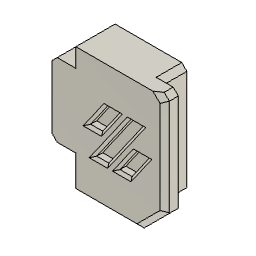
v0.2 Formbot Deck Chain Gap Cover v9 (Autodesk Fusion 360 design; units mm, degrees)
Autodesk Fusion 360 part; units mm, degrees
sketch "Base dimensions" plane through (0, 0, 0) normal (0, 1, 0) x (1, 0, 0)
  line L0 (-15, -8) -> (-6.6, -8)
  line L1 (-6.6, -8) -> (-6.6, 5)
  line L2 (-6.6, 5) -> (-15, 5)
  line L3 (-15, 5) -> (-15, -8)
  line L4 (-17.8, -5.8) -> (-15, -5.8)
  line L5 (-15, -5.8) -> (-15, 2.8)
  line L6 (-15, 2.8) -> (-17.8, 2.8)
  line L7 (-17.8, 2.8) -> (-17.8, -5.8)
  line L8 (-15.0127, 7) -> (-4.6, 7)
  line L9 (-4.6, 7) -> (-4.6, -8)
  line L10 (-4.6, -8) -> (-15.0127, -8)
  line L11 (-15.0127, -8) -> (-15.0127, 7)
  dimension "d1" = 8.4
  dimension "d2" = 13
  dimension "d3" = 2.2
  dimension "d4" = 2.2
  dimension "d5" = 2
  dimension "d6" = 2
  dimension "d21" = 2.8
  constraint horizontal L0
  constraint vertical L1
  constraint horizontal L2
  constraint vertical L3
  constraint horizontal L4
  constraint vertical L5
  constraint horizontal L6
  constraint vertical L7
  constraint coincident L3 L5.end
  constraint horizontal L8
  constraint vertical L9
  constraint horizontal L10
  constraint vertical L11
  measures "d1" distance of L0.start L0.end
  measures "d2" distance of L0.start L2.end
  measures "d3" distance of L0 L4
  measures "d4" distance of L2 L6
  measures "d5" distance of L0.end L9.end
  measures "d6" distance of L1.end L8
  measures "d21" distance of L3 L7
extrude "Extrude1" add sketch "Base dimensions" along normal blind 3 contours L0 L1 L2 L3 L5 L10 | L4 L6 L7 L11 makes body 1 at (-12.2, 0, 3.6667) makes body 2 at (-17.8, 1, 0.0667)
extrude "Extrude2" add sketch "Base dimensions" against normal blind 1.6 contours L0 L1 L2 L3 L5 L10 | L4 L6 L7 L11 bodies 1 2
extrude "Extrude3" add sketch "Base dimensions" against normal blind 1.6 contours L1 L2 L3 L6 L8 L9 L10 L11 bodies 1 2
chamfer "Chamfer1" distance 0.6 angle 45 6 edges at (-6.6, 1.5, -5) (-15, 1.5, -5) (-6.6, 1.5, 8) (-15, 0.7, 8) (-17.8, 0.7, 5.8) (-17.8, 0.7, -2.8) on bodies 1 2
chamfer "Chamfer2" distance 0.6 angle 45 3 edges at (-4.6, -0.8, 8) (-4.6, -0.8, -7) (-15.0127, -0.8, -7) on bodies 1
extrude "Extrude4" add 1 faces at (-15.9418, -1.6, 0.2667) along direction (0, -1, 0) blind 0.004 on bodies 1 bodies 1
extrude "Extrude5" cut 1 faces at (-15.9418, -1.604, 0.2667) along direction (0, 1, 0) up to surface (0.004 mm away) on bodies 1 bodies 1
chamfer "Chamfer3" distance 0.55 distance2 0.55 7 edges at (-14.7127, -1.6, -6.7) (-9.8064, -1.6, -7) (-4.9, -1.6, -6.7) (-4.6, -1.6, 0.5) (-4.9, -1.6, 7.7) (-9.8, -1.6, 8) (-14.7, -1.6, 7.7) measured on face at (-14.6127, -0.5333, -6.8) measured on face at (-8.0667, -1.6, -0.6) measured on face at (-5, -0.5333, -6.8) measured on face at (-8.0667, -1.6, -0.6) measured on face at (-4.8, -0.5333, 7.6) measured on face at (-8.0667, -1.6, -0.6) measured on face at (-14.6, -0.0667, 7.8) on bodies 1
delete_face "DeleteFace1" 1 faces at (-14.8, 1, -4.6) on bodies 1
delete_face "DeleteFace2" 1 faces at (-14.6, 0.3, 7.8) on bodies 1
delete_face "DeleteFace3" 1 faces at (-14.8, -1.0919, 7.5407) on bodies 1
delete_face "DeleteFace4" 1 faces at (-8.5426, -1.2333, 7.8167) on bodies 1
delete_face "DeleteFace5" 1 faces at (-4.8, -0.35, -6.6) on bodies 1
delete_face "DeleteFace6" 1 faces at (-5.0759, -1.2333, -6.6167) on bodies 1
chamfer "Chamfer4" distance 3 angle 45 1 edges at (-4.6, -0.525, -7) on bodies 1
chamfer "Chamfer5" distance 0.6 angle 45 1 edges at (-6.1, -1.6, -5.5) on bodies 1
delete_face "DeleteFace7" 1 faces at (-12.0894, -1.2333, -6.8167) on bodies 1
chamfer "Chamfer6" distance 0.6 angle 45 1 edges at (-11.0417, -1.6, -7) on bodies 1
sketch "Voron Logo" plane through (0, -1.6, 0) normal (0, -1, 0) x (1, 0, 0)
  line L0 (-14.2349, -6.4) -> (-7.8485, -6.4)
  line L1 (-7.8485, -6.4) -> (-5.15, -3.7015)
  line L2 (-5.15, -3.7015) -> (-5.15, 7.1722)
  line L3 (-5.15, 7.1722) -> (-5.9778, 8)
  line L4 (-5.9778, 8) -> (-15, 8)
  line L5 (-15, 8) -> (-15, -2.8)
  line L6 (-15, -2.8) -> (-15.0127, -2.8)
  line L7 (-15.0127, -2.8) -> (-15.0127, -5.6222)
  line L8 (-15.0127, -5.6222) -> (-14.2349, -6.4)
  line L9 (-6.9247, 3.8293) -> (-11.315, -2.4407)
  line L10 (-11.315, -2.4407) -> (-13.3484, -2.4407)
  line L11 (-6.2132, 0.9443) -> (-8.5834, -2.4407)
  line L12 (-8.9581, 3.8293) -> (-6.9247, 3.8293)
  line L13 (-14.0599, 0.4443) -> (-11.6897, 3.8293)
  line L14 (-8.2466, 0.9443) -> (-6.2132, 0.9443)
  line L15 (-10.1365, 3.5793) -> (-12.1566, 0.6943)
  line L16 (-11.5595, 3.5793) -> (-10.1365, 3.5793)
  line L17 (-12.1566, 0.6943) -> (-13.5796, 0.6943)
  line L18 (-11.4451, -2.1907) -> (-12.8681, -2.1907)
  line L19 (-9.6563, 3.8293) -> (-12.0265, 0.4443)
  line L20 (-11.6897, 3.8293) -> (-9.6563, 3.8293)
  line L21 (-8.7135, -2.1907) -> (-10.1365, -2.1907)
  line L22 (-6.6934, 0.6943) -> (-8.7135, -2.1907)
  line L23 (-12.0265, 0.4443) -> (-14.0599, 0.4443)
  line L24 (-13.5796, 0.6943) -> (-11.5595, 3.5793)
  line L25 (-8.8279, 3.5793) -> (-7.4049, 3.5793)
  line L26 (-10.1365, -2.1907) -> (-8.1164, 0.6943)
  line L27 (-8.1164, 0.6943) -> (-6.6934, 0.6943)
  line L28 (-8.5834, -2.4407) -> (-10.6168, -2.4407)
  line L29 (-7.4049, 3.5793) -> (-11.4451, -2.1907)
  line L30 (-12.8681, -2.1907) -> (-8.8279, 3.5793)
  line L31 (-13.3484, -2.4407) -> (-8.9581, 3.8293)
  line L32 (-10.6168, -2.4407) -> (-8.2466, 0.9443)
  point P0 (-15.3814, -7.6838)
  point P1 (-15.3814, 11.6728)
  point P2 (-15.3814, 9.1162)
extrude "Extrude9" add 1 faces at (-15, 0.4667, 4.4) along direction (-1, 0, 0) up to surface (0.0127 mm away) on bodies 1 bodies 1
extrude "Extrude6" cut sketch "Voron Logo" against normal blind 1 contours L15 L16 L17 L24 | L18 L25 L29 L30 | L21 L22 L26 L27 bodies 1
chamfer "Chamfer7" distance 0.3 angle 45 12 edges at (-7.7035, -1.6, -0.7482) (-7.4049, -1.6, 0.6943) (-9.1265, -1.6, -0.7482) (-9.425, -1.6, -2.1907) (-9.425, -1.6, 0.6943) (-12.1566, -1.6, -2.1907) (-10.848, -1.6, 0.6943) (-8.1164, -1.6, 3.5793) (-11.1466, -1.6, 2.1368) (-10.848, -1.6, 3.5793) (-12.5696, -1.6, 2.1368) (-12.8681, -1.6, 0.6943) on bodies 1
delete_face "DeleteFace8" 1 faces at (-14.7534, -1.4167, -6.1407) on bodies 1
delete_face "DeleteFace9" 1 faces at (-14.8127, -0.8667, -6.6) on bodies 1
chamfer "Chamfer8" distance 0.6 angle 45 1 edges at (-15.0127, -0.5, -7) on bodies 1
sketch "Sketch3" plane through (-17.8, 0, 0) normal (-1, 0, 0) x (0, -1, 0)
  line L0 (1.6, -2.2) -> (1.6, 5.2)
  line L1 (1.6, 5.2) -> (-3, 5.2)
  line L2 (-3, 5.2) -> (-3, -2.2)
  line L3 (-3, -2.2) -> (1.6, -2.2)
  line L4 (-3, 4.4) -> (0.4, 4.4)
  line L5 (0.4, 4.4) -> (0.4, -1.4)
  line L6 (0.4, -1.4) -> (-3, -1.4)
  line L7 (-3, -1.4) -> (-3, 4.4)
  line L8 (-3, -2.8) -> (1.6, -2.8)
  line L9 (-3, 8) -> (1.6, 8)
  line L10 (1.6, 5.8) -> (-3, 5.8)
  dimension "d29" = 1.4
  dimension "d31" = 1.2
  dimension "d32" = 1.4
  constraint horizontal L4
  constraint vertical L5
  constraint horizontal L6
  constraint vertical L7
  constraint coincident L2 L4.start
  measures "d29" distance of L6 L8
  measures "d31" distance of L0 L5
  measures "d32" distance of L4 L10
extrude "Extrude7" cut sketch "Sketch3" against normal blind 1 contours L2 L4 L5 L6 L7 bodies 1
chamfer "Chamfer9" distance 0.4 angle 45 2 edges at (-17.8, 1.3, -1.4) (-17.8, 1.3, 4.4) on bodies 1
chamfer "Chamfer10" distance 0.4 angle 45 1 edges at (-17.8, -0.4, 1.5) on bodies 1
equation "d1 = 11.2 mm - 2.8 mm"
